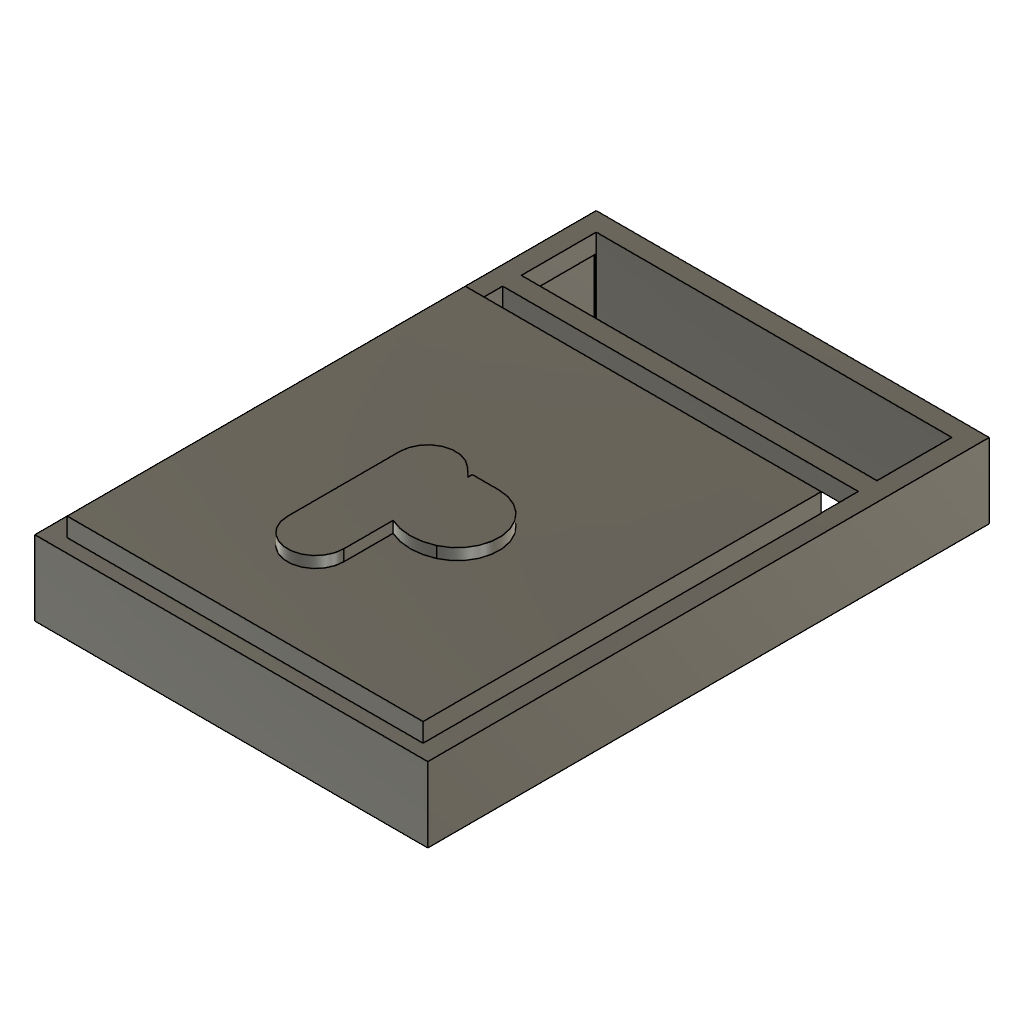
Untitled (Autodesk Fusion 360 design; units mm, degrees)
part number: 2026-10-04-11-00-03-890
part number: 2026-10-04-11-17-13-789
Autodesk Fusion 360 part; units mm, degrees
sketch "Sketch1" plane through (0, 0, 0) normal (0, 0, 1) x (1, 0, 0)
  line L0 (-25, 50) -> (80, 50)
  line L1 (80, 50) -> (80, -100)
  line L2 (80, -100) -> (-25, -100)
  line L3 (-25, -100) -> (-25, 50)
  line L4 (-20, 45) -> (75, 45)
  line L5 (75, 45) -> (75, 25)
  line L6 (75, 25) -> (-20, 25)
  line L7 (-20, 25) -> (-20, 45)
  line L8 (-20, 20) -> (75, 20)
  line L9 (75, 20) -> (75, 10)
  line L10 (75, 10) -> (-20, 10)
  line L11 (-20, 10) -> (-20, 20)
  dimension "d1" = 105
  dimension "d2" = 150
  constraint horizontal L0
  constraint vertical L1
  constraint horizontal L2
  constraint vertical L3
  constraint horizontal L4
  constraint vertical L5
  constraint horizontal L6
  constraint vertical L7
  constraint horizontal L8
  constraint vertical L9
  constraint horizontal L10
  constraint vertical L11
  measures "d1" distance of L0.start L0.end
  measures "d2" distance of L0.start L2.end
extrude "Extrude1" add sketch "Sketch1" along normal blind 20 makes body 1
sketch "Sketch2" plane through (0, 0, 0) normal (0, 0, 1) x (1, 0, 0)
  line L0 (-20.26, 44.7118) -> (75.3115, 44.7118)
  line L1 (75.3115, 44.7118) -> (75.3115, -94.4537)
  line L2 (75.3115, -94.4537) -> (-20.26, -94.4537)
  line L3 (-20.26, -94.4537) -> (-20.26, 44.7118)
  constraint horizontal L0
  constraint vertical L1
  constraint horizontal L2
  constraint vertical L3
extrude "Extrude2" cut sketch "Sketch2" along normal blind 15 bodies 1
sketch "Sketch3" plane through (0, 0, 0) normal (0, 0, 1) x (1, 0, 0)
  circle A0 centre (70, 0) radius 2.5
  circle A1 centre (-10, 0) radius 2.5
  circle A2 centre (70, -90) radius 2.5
  circle A3 centre (-10, -90) radius 2.5
  circle A4 centre (50, 0) radius 2.5
  circle A5 centre (50, -20) radius 2.5
  circle A6 centre (70, -20) radius 2.5
  circle A7 centre (10, 0) radius 2.5
  circle A8 centre (-10, -20) radius 2.5
  circle A9 centre (10, -20) radius 2.5
  circle A10 centre (30, 0) radius 2.5
  circle A11 centre (30, -20) radius 2.5
  dimension "d7" = 5
  dimension "d8" = 5
  dimension "d9" = 5
  dimension "d10" = 5
  dimension "d11" = 5
  dimension "d12" = 5
  dimension "d13" = 5
  dimension "d14" = 5
  dimension "d15" = 5
  dimension "d16" = 5
  dimension "d17" = 5
  dimension "d18" = 5
  measures "d7" diameter of A0
  measures "d8" diameter of A1
  measures "d9" diameter of A2
  measures "d10" diameter of A3
  measures "d11" diameter of A4
  measures "d12" diameter of A5
  measures "d13" diameter of A6
  measures "d14" diameter of A7
  measures "d15" diameter of A8
  measures "d16" diameter of A9
  measures "d17" diameter of A10
  measures "d18" diameter of A11
extrude "Extrude3" cut sketch "Sketch3" along normal blind 40 bodies 1
thread "Thread1" "ISO Metric profile 5.0 M5x0.8 M5x0.8 6H" major diameter 5.12 minor diameter 4.234 pitch 0.8 angle 60 resizes the face on face at (72.4969, -19.8754, 16.6667) on bodies 1
thread "Thread2" "ISO Metric profile 5.0 M5x0.8 M5x0.8 6H" major diameter 5.12 minor diameter 4.234 pitch 0.8 angle 60 resizes the face on face at (52.4969, -19.8754, 16.6667) on bodies 1
thread "Thread3" "ISO Metric profile 5.0 M5x0.8 M5x0.8 6H" major diameter 5.12 minor diameter 4.234 pitch 0.8 angle 60 resizes the face on face at (32.4969, -19.8754, 16.6667) on bodies 1
thread "Thread4" "ISO Metric profile 5.0 M5x0.8 M5x0.8 6H" major diameter 5.12 minor diameter 4.234 pitch 0.8 angle 60 resizes the face on face at (32.4876, 0.2489, 18.3333) on bodies 1
thread "Thread5" "ISO Metric profile 5.0 M5x0.8 M5x0.8 6H" major diameter 5.12 minor diameter 4.234 pitch 0.8 angle 60 resizes the face on face at (12.4876, 0.2489, 18.3333) on bodies 1
thread "Thread6" "ISO Metric profile 5.0 M5x0.8 M5x0.8 6H" major diameter 5.12 minor diameter 4.234 pitch 0.8 angle 60 resizes the face on face at (-7.5124, 0.2489, 18.3333) on bodies 1
thread "Thread7" "ISO Metric profile 5.0 M5x0.8 M5x0.8 6H" major diameter 5.12 minor diameter 4.234 pitch 0.8 angle 60 resizes the face on face at (-7.5031, -19.8754, 16.6667) on bodies 1
thread "Thread8" "ISO Metric profile 5.0 M5x0.8 M5x0.8 6H" major diameter 5.12 minor diameter 4.234 pitch 0.8 angle 60 resizes the face on face at (12.4969, -19.8754, 16.6667) on bodies 1
thread "Thread9" "ISO Metric profile 5.0 M5x0.8 M5x0.8 6H" major diameter 5.12 minor diameter 4.234 pitch 0.8 angle 60 resizes the face on face at (52.4876, 0.2489, 18.3333) on bodies 1
thread "Thread10" "ISO Metric profile 5.0 M5x0.8 M5x0.8 6H" major diameter 5.12 minor diameter 4.234 pitch 0.8 angle 60 resizes the face on face at (72.4876, 0.2489, 18.3333) on bodies 1
thread "Thread11" "ISO Metric profile 5.0 M5x0.8 M5x0.8 6H" major diameter 5.12 minor diameter 4.234 pitch 0.8 angle 60 resizes the face on face at (67.6508, -89.1449, 18.3333) on bodies 1
thread "Thread12" "ISO Metric profile 5.0 M5x0.8 M5x0.8 6H" major diameter 5.12 minor diameter 4.234 pitch 0.8 angle 60 resizes the face on face at (-12.3492, -89.1449, 18.3333) on bodies 1
sketch "Sketch4" plane through (0, 0, 0) normal (0, 0, 1) x (1, 0, 0)
  line L0 (-20, 10) -> (75.1056, 10)
  line L1 (75.1056, 10) -> (75.1056, -96.3646)
  line L2 (75.1056, -96.3646) -> (-20, -96.3646)
  line L3 (-20, -96.3646) -> (-20, 10)
  constraint horizontal L0
  constraint vertical L1
  constraint horizontal L2
  constraint vertical L3
extrude "Extrude1'" add sketch "Sketch4" along normal blind 10 separate body makes body 2 in component "Component"
move_body "Move1" bodies 2 to x (1, 0, 0) y (0, 1, 0) z (0, 0, 1) at (0, 0, 20) in component "Component"
extrude "Extrude2'" cut 1 faces at (43.4037, -60.9097, 30) along direction (0, 0, -1) blind 5 on bodies 2 bodies 2 in component "Component"
combine "Combine1" operation add target body 1 tool bodies 2
sketch "Sketch5" plane through (0, 0, 25) normal (0, 0, 1) x (-1, 0, 0)
  line L0 (20, 96.3646) -> (-75.1056, 96.3646)
  line L1 (-75.1056, 96.3646) -> (-75.1056, -10)
  line L2 (-75.1056, -10) -> (20, -10)
  line L3 (20, -10) -> (20, 96.3646)
  circle A0 centre (-20, 40) radius 7.5
  line L4 (-12.5, 40) -> (-12.5, 70)
  arc A1 (-12.5, 70) -> (-27.5528, 70) centre (-20.0264, 70) ccw
  line L5 (-27.5528, 70) -> (-27.5528, 36.787)
  line L6 (-27.5528, 36.787) -> (-25.1136, 34.5135)
  line L7 (-27.5528, 35.6503) -> (-34.6305, 35.6503)
  arc A2 (-39.1972, 56.8295) -> (-34.6305, 35.6503) centre (-34.6305, 46.7322) ccw
  arc A3 (-27.5528, 56.8295) -> (-39.1972, 56.8295) centre (-33.375, 43.9561) ccw
  line L8 (-27.5528, 36.787) -> (-27.5528, 56.8295)
  line L9 (-27.5528, 56.8295) -> (-27.5528, 35.6503)
  dimension "d49" = 15
  constraint coincident A0 L4.start
  constraint tangent A0 L4
  constraint perpendicular L0 L4
  constraint tangent L4 A1
  constraint coincident A0 L6.end
  constraint tangent A0 L6
  constraint coincident L5 L7.start
  constraint perpendicular L5 L7
  constraint perpendicular L1 L7
  constraint tangent L7 A2
  constraint coincident L5 A3.start
  constraint tangent A2 A3
  measures "d49" diameter of A0
extrude "Extrude4" add sketch "Sketch5" along normal blind 3 contours A0 | A0 L4 A1 L5 L6 L8 L9 | L5 L7 A2 A3 L8 L9 bodies 1
component "Component" placed x (1, 0, 0) y (0, 1, 0) z (0, 0, 1) at (0, 0, 0)
